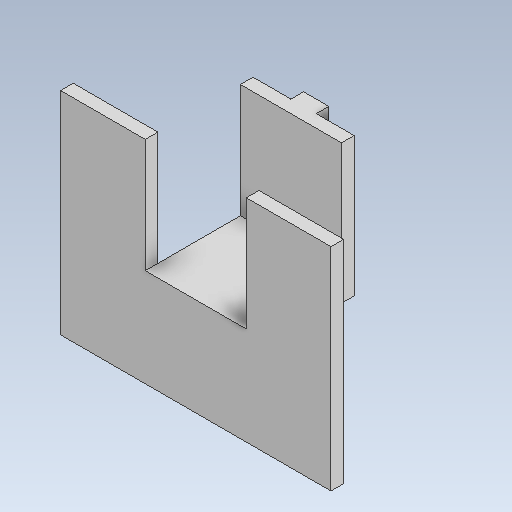
# Autodesk Inventor part: center_tray
Saved by Autodesk Inventor 2020 (Build 240168000, 168)
## iProperties
Created: 2022-09-22
Part Number: center_tray
Material: 일반
Document SubType Name: Modeling
Designer: SeungJin
Density: 1 g/cm^3
Appearance: 기본값
Author: SeungJin
Autodesk Inventor part; units mm, degrees
ref_plane "YZ Plane" through (0, 0, 0) normal (1, 0, 0) x (0, 1, 0)
ref_plane "XZ Plane" through (0, 0, 0) normal (0, 1, 0) x (-1, 0, 0)
ref_plane "XY Plane" through (0, 0, 0) normal (0, 0, 1) x (1, 0, 0)
sketch "스케치1" plane through (0, 0, 0) normal (0, 0, 1) x (1, 0, 0)
  line L0 (0, -188.5) -> (0, 261.5) projected
  line L1 (20, -188.5) -> (20, 261.5) projected
  line L2 (-30, -188.5) -> (-30, 261.5) projected
  line L3 (50, -188.5) -> (50, 261.5) projected
  line L4 (195.5, 192.5) -> (-175.5, 192.5) projected
  line L5 (-30, 167.5) -> (-107, 167.5) projected
  line L6 (50, 167.5) -> (127, 167.5) projected
  line L7 (280, 30) -> (-260, 30) projected
  line L8 (-30, 167.5) -> (50, 167.5)
  line L9 (-145.5, 0) -> (165.5, 0) projected
  line L10 (-30, 57.5) -> (50, 57.5)
  point P0 (0, 0)
  point P1 (-30, 0)
  point P2 (50, 0)
  point P3 (-30, 30)
  point P4 (50, 30)
  dimension "d10" = 27.5
  constraints: 4 end point, 2 point on line, 1 collinear, 1 perpendicular
  measures "d10" distance between parallel lines of L7 L10
extrude "돌출1" add sketch "스케치1" along normal blind 10 contours L10 L2 L8 L0 | L0 L8 L1 L10 | L1 L8 L3 L10
sketch "스케치2" plane through (0, 0, 10) normal (0, 0, 1) x (1, 0, 0)
  line L0 (0, -188.5) -> (0, 261.5) projected
  line L1 (20, -188.5) -> (20, 261.5) projected
  line L2 (50, 57.5) -> (50, 167.5) projected
  line L3 (50, 167.5) -> (-30, 167.5) projected
  line L4 (-30, 167.5) -> (-30, 57.5) projected
  line L5 (-30, 167.5) -> (-30, 30) projected
  line L6 (-30, 77.5) -> (50, 77.5)
  line L7 (50, 30) -> (50, 167.5) projected
  line L8 (-30, 57.5) -> (50, 57.5)
  line L9 (-30, 57.5) -> (50, 57.5) projected
  point P0 (0, 0)
  point P1 (-30, 0)
  point P2 (50, 0)
  point P3 (20, 77.5)
  point P4 (0, 77.5)
  dimension "d2" = 90
  dimension "d7" = 20
  constraints: 4 end point, 4 point on line, 2 perpendicular
  measures "d2" distance between parallel lines of L3 L6
  measures "d7" distance between parallel lines of L6 L8
ref_plane "작업 평면1" through (-97, 10, 75.3) normal (0, 0, -1) x (0, 1, 0)
extrude "돌출2" add sketch "스케치2" along normal up to surface (65.3 mm away) contours L8 L4 L6 L0 | L0 L6 L1 L8 | L1 L6 L2 L8
sketch "스케치3" plane through (0, 77.5, 75.3) normal (0, 0, 1) x (1, 0, 0)
  line L0 (50, 0) -> (-30, 0) projected
  line L1 (-107, 90) -> (-107, -77.5) projected
  line L2 (-30, 0) -> (-30, 90) projected
  line L3 (-30, 90) -> (-107, 90) projected
  line L4 (127, 90) -> (127, -77.5) projected
  line L5 (50, 90) -> (127, 90) projected
  line L6 (50, -77.5) -> (50, 90) projected
  line L7 (127, -77.5) -> (50, -77.5) projected
  line L8 (50, 90) -> (-30, 90) projected
  line L9 (-145.5, -77.5) -> (165.5, -77.5) projected
  line L10 (-30, 90) -> (-30, 0) projected
  line L11 (-30, 0) -> (0, 0)
  line L12 (50, 0) -> (0, 0) projected
  line L13 (20, 0) -> (50, 0)
  line L14 (-30, 0) -> (-30, -20) projected
  line L15 (-30, -20) -> (50, -20) projected
  line L16 (50, -20) -> (50, 0) projected
  line L17 (-97, -67.5) -> (-97, 90) projected
  line L18 (117, -67.5) -> (117, 90) projected
  line L19 (-97, -67.5) -> (-97, -77.5)
  line L20 (117, -67.5) -> (117, -77.5)
  point P0 (0, -77.5)
  point P1 (0, -77.5)
  point P2 (20, -77.5)
  constraints: 8 end point, 3 point on line, 1 parallel, 1 perpendicular, 1 vertical, 3 other
extrude "돌출3" add sketch "스케치3" along normal blind 10 contours L6 L15 L14 L0 | L6 L5 L18 L20 L7 | L6 L9 L19 L17 L3 L2 L14 L15
sketch "스케치4" plane through (0, 0, 0) normal (0, 0, -1) x (-1, 0, 0)
  line L0 (0, -188.5) -> (0, 261.5) projected
  line L1 (-20, -188.5) -> (-20, 261.5) projected
  line L2 (-280, 30) -> (260, 30) projected
  line L3 (-280, 198.5399) -> (260, 198.5399) projected
  line L4 (175.5, 192.5) -> (30, 192.5) projected
  line L5 (30, 167.5) -> (30, 57.5) projected
  line L6 (-50, 167.5) -> (30, 167.5) projected
  line L7 (-50, 57.5) -> (-50, 167.5) projected
  line L8 (30, 57.5) -> (-50, 57.5) projected
  point P0 (0, 0)
  point P1 (0, 167.5)
  point P2 (-20, 167.5)
  point P3 (-20, 30)
  point P4 (0, 30)
  point P5 (-20, 57.5)
  point P6 (0, 57.5)
extrude "돌출4" add sketch "스케치4" along normal blind 10 contours L8 L1 L6 L0
